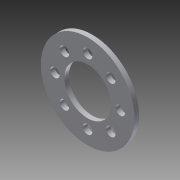
# Autodesk Inventor part: 8
Saved by Autodesk Inventor 2013 (Build 170138000, 138)
## iProperties
Created: 2014-03-29
Part Number: 8
Material: アセタール樹脂、白
Document SubType Name: Modeling
Designer: andou
Density: 1 g/cm^3
Author: andou
Title: Horn-Spacer
Autodesk Inventor part; units mm, degrees
ref_plane "YZ Plane" through (0, 0, 0) normal (1, 0, 0) x (0, 1, 0)
ref_plane "XZ Plane" through (0, 0, 0) normal (0, 1, 0) x (-1, 0, 0)
ref_plane "XY Plane" through (0, 0, 0) normal (0, 0, 1) x (1, 0, 0)
sketch "スケッチ1" plane through (0, 0, 0) normal (0, 1, 0) x (-1, 0, 0)
  circle A0 centre (0, 0) radius 10
  circle A1 centre (0, 0) radius 5
  dimension "d0" = 20
  dimension "d2" = 10
  constraints: 2 centre point, 2 coincident
  measures "d0" diameter of A0
  measures "d2" diameter of A1
extrude "押し出し1" add sketch "スケッチ1" along normal blind 1
sketch "スケッチ2" plane through (0, 1, 0) normal (0, 1, 0) x (1, 0, 0)
  circle A0 centre (0, 0) radius 5 projected
  circle A1 centre (0, 7) radius 1
  dimension "d5" = 2
  dimension "d7" = 7
  dimension "d8" = 0
  constraints: 1 centre point
  measures "d5" diameter of A1
  measures "d7" distance of A1.centre A0.centre
  measures "d8" horizontal distance of A1.centre A0.centre
hole "穴1" at (0, 1, -7) direction (0, -1, 0) diameter 2 end through all
pattern_circular "円形状パターン1" count 8 over 360 about axis through (0, 0, 0) along (0, 1, 0) of "穴1"
